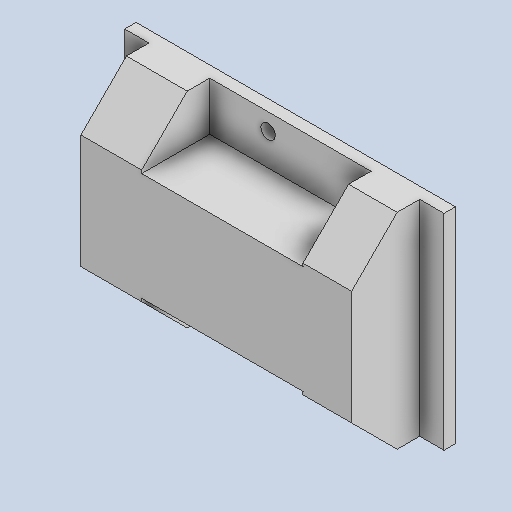
# Autodesk Inventor part: FuseBox_04980933.X
Saved by Autodesk Inventor 2022 (Build 260153000, 153)
## iProperties
Created: 2021-02-16
Part Number: FuseBox_04980933.X
Material: Generic
Document SubType Name: Modeling
Designer: Viktor
Density: 1 g/cm^3
Appearance: Default
Author: Viktor
Autodesk Inventor part; units mm, degrees
ref_plane "YZ Plane" through (0, 0, 0) normal (1, 0, 0) x (0, 1, 0)
ref_plane "XZ Plane" through (0, 0, 0) normal (0, 1, 0) x (-1, 0, 0)
ref_plane "XY Plane" through (0, 0, 0) normal (0, 0, 1) x (1, 0, 0)
sketch "Sketch1" plane through (0, 0, 0) normal (0, 0, 1) x (1, 0, 0)
  line L0 (-65.675, -42.2) -> (65.675, -42.2)
  line L1 (65.675, -42.2) -> (65.675, 42.2)
  line L2 (65.675, 42.2) -> (-65.675, 42.2)
  line L3 (-65.675, 42.2) -> (-65.675, -42.2)
  line L4 (-65.675, -42.2) -> (65.675, 42.2) construction
  line L5 (65.675, -42.2) -> (-65.675, 42.2) construction
  point P0 (0, 0)
  dimension "d0" = 131.35
  dimension "d1" = 84.4
  constraints: 12 end point, 2 midpoint, 2 parallel, 1 horizontal, 1 perpendicular
  measures "d0" distance between parallel lines of L1 L3
  measures "d1" distance of L0.end L1.end
extrude "Extrusion1" add sketch "Sketch1" along normal blind 32.7
sketch "Sketch2" plane through (0, 0, 32.7) normal (0, 0, 1) x (1, 0, 0)
  line L0 (65.675, 42.2) -> (-65.675, 42.2) projected
  line L1 (-65.675, -42.2) -> (65.675, -42.2) projected
  line L2 (-30.675, 42.2) -> (35.675, 42.2)
  line L3 (35.675, 42.2) -> (35.675, 22.2)
  line L4 (35.675, 22.2) -> (-30.675, 22.2)
  line L5 (-30.675, 22.2) -> (-30.675, 42.2)
  line L6 (-30.675, -42.2) -> (35.675, -42.2)
  line L7 (35.675, -42.2) -> (35.675, -22.2)
  line L8 (35.675, -22.2) -> (-30.675, -22.2)
  line L9 (-30.675, -22.2) -> (-30.675, -42.2)
  line L10 (65.675, -42.2) -> (65.675, 42.2) projected
  line L11 (-65.675, 42.2) -> (-65.675, -42.2) projected
  line L12 (65.675, 42.2) -> (55.675, 42.2)
  line L13 (55.675, 42.2) -> (55.675, -42.2)
  line L14 (55.675, -42.2) -> (65.675, -42.2)
  line L15 (65.675, -42.2) -> (65.675, 42.2)
  line L16 (-65.675, 42.2) -> (-55.675, 42.2)
  line L17 (-55.675, 42.2) -> (-55.675, -42.2)
  line L18 (-55.675, -42.2) -> (-65.675, -42.2)
  line L19 (-65.675, -42.2) -> (-65.675, 42.2)
  point P0 (0, 0)
  dimension "d5" = 20
  dimension "d6" = 20
  dimension "d7" = 30
  dimension "d8" = 35
  dimension "d9" = 35
  dimension "d10" = 10
  dimension "d11" = 10
  constraints: 32 end point, 8 parallel, 5 point on line, 4 horizontal, 4 perpendicular
  measures "d5" distance between parallel lines of L0 L4
  measures "d6" distance between parallel lines of L1 L8
  measures "d7" distance between parallel lines of L10 L3
  measures "d8" distance between parallel lines of L11 L5
  measures "d9" distance between parallel lines of L11 L9
  measures "d10" distance between parallel lines of L19 L17
  measures "d11" distance between parallel lines of L10 L13
extrude "Extrusion2" cut sketch "Sketch2" against normal blind 28 contours L10 L1 L13 L0 | L3 L4 L5 L0 | L1 L9 L8 L7 | L17 L1 L11 L0
chamfer "Chamfer1" distance 18.75 angle 45 4 edges at (-43.175, -42.2, 32.7) (45.675, -42.2, 32.7) (45.675, 42.2, 32.7) (-43.175, 42.2, 32.7)
sketch "Sketch3" plane through (0, 0, 4.7) normal (0, 0, 1) x (1, 0, 0)
  circle A0 centre (-6.675, 35.2) radius 3
  circle A1 centre (-10.675, -35.2) radius 3
  circle A2 centre (13.325, -35.2) radius 3
  line L0 (-30.675, 42.2) -> (35.675, 42.2) projected
  line L1 (35.675, -42.2) -> (55.675, -42.2) projected
  line L2 (-65.675, -42.2) -> (-65.675, 42.2) projected
  point P0 (0, 0)
  dimension "d17" = 24
  dimension "d18" = 20
  dimension "d19" = 70.4
  dimension "d20" = 7
  dimension "d21" = 84.4
  dimension "d22" = 6
  dimension "d23" = 6
  dimension "d24" = 6
  dimension "d25" = 55
  dimension "d26" = 0
  constraints: 3 centre point
  measures "d17" distance of A2.centre A1.centre
  measures "d18" horizontal distance of A0.centre A2.centre
  measures "d19" vertical distance of A1.centre A0.centre
  measures "d20" distance from line of L0 A0.centre
  measures "d21" distance between parallel lines of L1 L0
  measures "d22" diameter of A0
  measures "d23" diameter of A1
  measures "d24" diameter of A2
  measures "d25" distance from line of L2 A1.centre
  measures "d26" vertical distance of A1.centre A2.centre
extrude "Extrusion3" cut sketch "Sketch3" against normal blind 28
equation "\"d6\" = d5"
equation "\"d9\" = d8"
equation "\"d20\" = -0.5 * d19 + 0.5 * d21"
equation "\"d23\" = d22"
equation "\"d24\" = d22"
body "Solid1"
